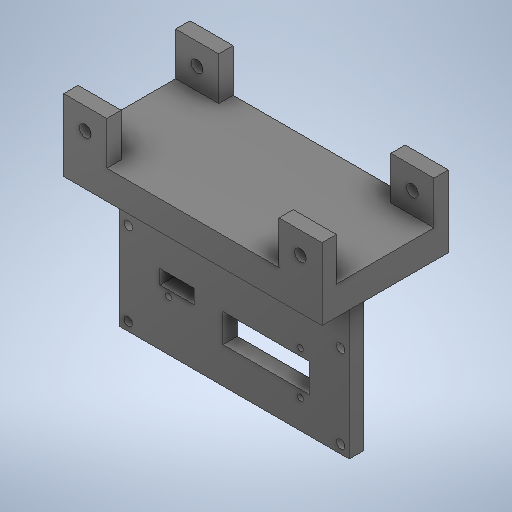
# Autodesk Inventor part: rail_top
Saved by Autodesk Inventor 2026.2 (Build 302298010, 298A)
## iProperties
Created: 2026-05-03
Part Number: rail_top
Material: ABS Plastic
Document SubType Name: Modeling
Designer: chris
Density: 1.06 g/cm^3
Appearance: Smooth - White
Author: chris
Autodesk Inventor part; units mm, degrees
ref_plane "YZ Plane" through (0, 0, 0) normal (1, 0, 0) x (0, 1, 0)
ref_plane "XZ Plane" through (0, 0, 0) normal (0, 1, 0) x (-1, 0, 0)
ref_plane "XY Plane" through (0, 0, 0) normal (0, 0, 1) x (1, 0, 0)
sketch "Sketch1" plane through (0, 0, 0) normal (0, 1, 0) x (-1, 0, 0)
  line L0 (45, 22) -> (-45, 22)
  line L1 (-45, 22) -> (-45, -22)
  line L2 (-45, -22) -> (45, -22)
  line L3 (45, -22) -> (45, 22)
  line L4 (45, 22) -> (-45, -22) construction
  line L5 (-45, 22) -> (45, -22) construction
  point P0 (0, 0)
  dimension "d0" = 90
  dimension "d1" = 44
  constraints: 12 end point, 2 midpoint, 2 parallel, 1 horizontal, 1 perpendicular
  measures "d0" distance of L2.end L1.end
  measures "d1" distance of L1.end L0.end
extrude "Extrusion1" add sketch "Sketch1" along normal blind 10
sketch "Sketch2" plane through (0, 10, 0) normal (0, 1, 0) x (1, 0, 0)
  line L0 (45, -22) -> (30, -22)
  line L1 (30, -22) -> (30, -17)
  line L2 (30, -17) -> (45, -17)
  line L3 (45, -17) -> (45, -22)
  line L4 (45, 17) -> (30, 17)
  line L5 (30, 17) -> (30, 22)
  line L6 (30, 22) -> (45, 22)
  line L7 (45, 22) -> (45, 17)
  line L8 (-45, -22) -> (-30, -22)
  line L9 (-30, -22) -> (-30, -17)
  line L10 (-30, -17) -> (-45, -17)
  line L11 (-45, -17) -> (-45, -22)
  line L12 (-45, 17) -> (-30, 17)
  line L13 (-30, 17) -> (-30, 22)
  line L14 (-30, 22) -> (-45, 22)
  line L15 (-45, 22) -> (-45, 17)
  line L16 (-45, 22) -> (-45, -22) projected
  line L17 (-45, -22) -> (45, -22) projected
  line L18 (45, 22) -> (-45, 22) projected
  line L19 (45, -22) -> (45, 22) projected
  point P0 (0, 0)
  dimension "d4" = 5
  dimension "d5" = 5
  dimension "d6" = 5
  dimension "d7" = 5
  dimension "d8" = 15
  dimension "d9" = 15
  dimension "d10" = 15
  dimension "d11" = 15
  constraints: 32 end point, 8 collinear, 8 parallel, 4 horizontal, 4 perpendicular
  measures "d4" distance of L2.end L0.start
  measures "d5" distance of L6.end L4.start
  measures "d6" distance of L12.end L13.end
  measures "d7" distance of L8.end L9.end
  measures "d8" distance of L0.start L0.end
  measures "d9" distance of L5.end L6.end
  measures "d10" distance of L12.start L12.end
  measures "d11" distance of L9.end L10.end
extrude "Extrusion2" add sketch "Sketch2" along normal blind 15 contours L0 L1 L2 L3 | L8 L11 L10 L9 | L4 L5 L6 L7 | L15 L14 L13 L12
sketch "Sketch3" plane through (-45, 0, 22) normal (0, 0, 1) x (1, 0, 0)
  circle A0 centre (82.5, 17.5) radius 2.05
  circle A1 centre (7.5, 17.5) radius 2.05
  line L0 (75, 25) -> (90, 25) projected
  line L1 (90, 0) -> (90, 25) projected
  line L2 (0, 25) -> (15, 25) projected
  line L3 (15, 10) -> (15, 25) projected
  point P0 (45, 0)
  point P1 (15, 17.5)
  dimension "d14" = 4.1
  dimension "d15" = 4.1
  dimension "d16" = 7.5
  dimension "d17" = 7.5
  dimension "d18" = 7.5
  dimension "d19" = 7.5
  constraints: 2 centre point, 1 midpoint
  measures "d14" diameter of A0
  measures "d15" diameter of A1
  measures "d16" distance from line of L0 A0.centre
  measures "d17" distance from line of L1 A0.centre
  measures "d18" distance from line of L2 A1.centre
  measures "d19" distance of point (15, 17.5) A1.centre
extrude "Extrusion3" cut sketch "Sketch3" against normal through all
sketch "Sketch6" plane through (0, 0, 0) normal (0, -1, 0) x (1, 0, 0)
  line L0 (-7.5, -7.5) -> (7.5, -7.5)
  line L1 (7.5, -7.5) -> (7.5, 7.5)
  line L2 (7.5, 7.5) -> (-7.5, 7.5)
  line L3 (-7.5, 7.5) -> (-7.5, -7.5)
  line L4 (-7.5, -7.5) -> (7.5, 7.5) construction
  line L5 (7.5, -7.5) -> (-7.5, 7.5) construction
  point P0 (0, 0)
  dimension "d27" = 15
  dimension "d28" = 15
  constraints: 12 end point, 2 midpoint, 2 parallel, 1 horizontal, 1 perpendicular
  measures "d27" distance of L2.end L1.end
  measures "d28" distance of L1.end L0.end
extrude "Extrusion5" add sketch "Sketch6" along normal blind 15
sketch "Sketch7" plane through (7.5, 0, -7.5) normal (0, 0, -1) x (-1, 0, 0)
  circle A0 centre (7.5, -7.5) radius 4.5
  line L0 (-37.5, 0) -> (52.5, 0) projected
  line L1 (0, 0) -> (0, -15) projected
  point P0 (7.5, 0)
  dimension "d31" = 9
  dimension "d32" = 7.5
  dimension "d33" = 7.5
  constraints: 1 centre point
  measures "d31" diameter of A0
  measures "d32" distance from line of A0.centre L0
  measures "d33" distance from line of L1 A0.centre
extrude "Extrusion6" cut sketch "Sketch7" against normal through all
sketch "Sketch8" plane through (-7.5, 0, 7.5) normal (0, 0, 1) x (1, 0, 0)
  line L0 (47.5, 0) -> (-32.5, 0)
  line L1 (-32.5, 0) -> (-32.5, -50)
  line L2 (-32.5, -50) -> (47.5, -50)
  line L3 (47.5, -50) -> (47.5, 0)
  line L4 (-37.5, 0) -> (52.5, 0) projected
  line L5 (0, 0) -> (0, -15) projected
  line L6 (15, -15) -> (0, -15) projected
  line L7 (15, 0) -> (15, -15) projected
  circle A0 centre (7.5, -7.5) radius 4.5 projected
  line L8 (0, 0) -> (15, 0) projected
  line L9 (0, 0) -> (0, -15) projected
  line L10 (15, -15) -> (0, -15) projected
  line L11 (15, 0) -> (15, -15) projected
  point P0 (7.5, 0)
  point P1 (7.5, 0)
  dimension "d36" = 50
  dimension "d37" = 80
  dimension "d38" = 40
  constraints: 8 end point, 2 parallel, 1 collinear, 1 horizontal, 1 midpoint, 1 perpendicular
  measures "d36" distance of L0.end L1.end
  measures "d37" distance of L1.end L2.end
  measures "d38" distance from line of point (7.5, 0) L1
extrude "Extrusion7" add sketch "Sketch8" against normal blind 5 contours L3 L2 L1 L0 L5 L6 L7
sketch "Sketch10" plane through (-7.5, 0, 2.5) normal (0, 0, -1) x (-1, 0, 0)
  circle A0 centre (29.5, -47) radius 1.5
  circle A1 centre (-44.5, -47) radius 1.5
  circle A2 centre (29.5, -18) radius 1.5
  circle A3 centre (-44.5, -18) radius 1.5
  line L0 (-47.5, -50) -> (32.5, -50) projected
  line L1 (-47.5, 0) -> (-47.5, -50) projected
  line L2 (32.5, -50) -> (32.5, 0) projected
  point P0 (-7.5, 0)
  dimension "d58" = 3
  dimension "d59" = 3
  dimension "d60" = 3
  dimension "d61" = 3
  dimension "d62" = 3
  dimension "d63" = 3
  dimension "d64" = 3
  dimension "d65" = 3
  dimension "d66" = 29
  dimension "d67" = 29
  dimension "d68" = 3
  dimension "d69" = 3
  constraints: 4 centre point
  measures "d58" diameter of A0
  measures "d59" diameter of A1
  measures "d60" diameter of A2
  measures "d61" diameter of A3
  measures "d62" distance from line of L0 A1.centre
  measures "d63" distance from line of L1 A1.centre
  measures "d64" distance from line of A0.centre L0
  measures "d65" distance from line of L2 A0.centre
  measures "d66" distance of A3.centre A1.centre
  measures "d67" distance of A2.centre A0.centre
  measures "d68" distance from line of L1 A3.centre
  measures "d69" distance from line of L2 A2.centre
extrude "Extrusion9" cut sketch "Sketch10" against normal blind 5
sketch "Sketch11" plane through (-7.5, 0, 2.5) normal (0, 0, -1) x (-1, 0, 0)
  circle A0 centre (-30.5, -40) radius 1.05
  circle A1 centre (15.5, -32.5) radius 1.05
  circle A2 centre (-30.5, -25) radius 1.05
  line L0 (-47.5, 0) -> (-47.5, -50) projected
  line L1 (-47.5, -50) -> (32.5, -50) projected
  point P0 (-7.5, 0)
  dimension "d75" = 2.1
  dimension "d76" = 2.1
  dimension "d77" = 2.1
  dimension "d78" = 46
  dimension "d79" = 7.5
  dimension "d80" = 7.5
  dimension "d81" = 17
  dimension "d82" = 0
  dimension "d83" = 10
  constraints: 3 centre point
  measures "d75" diameter of A0
  measures "d76" diameter of A1
  measures "d77" diameter of A2
  measures "d78" horizontal distance of A1.centre A0.centre
  measures "d79" vertical distance of A1.centre A0.centre
  measures "d80" vertical distance of A1.centre A2.centre
  measures "d81" distance from line of L0 A0.centre
  measures "d82" horizontal distance of A0.centre A2.centre
  measures "d83" distance from line of L1 A0.centre
extrude "Extrusion10" cut sketch "Sketch11" against normal through all
sketch "Sketch12" plane through (-7.5, 0, 2.5) normal (0, 0, -1) x (-1, 0, 0)
  line L0 (-3.5, -37.5) -> (-33.5, -37.5)
  line L1 (-33.5, -37.5) -> (-33.5, -27.5)
  line L2 (-33.5, -27.5) -> (-3.5, -27.5)
  line L3 (-3.5, -27.5) -> (-3.5, -37.5)
  line L4 (0, -15) -> (-15, -15) projected
  line L5 (-47.5, 0) -> (-47.5, -50) projected
  point P0 (-7.5, 0)
  dimension "d86" = 30
  dimension "d87" = 10
  dimension "d88" = 12.5
  dimension "d89" = 14
  constraints: 8 end point, 2 parallel, 1 horizontal, 1 perpendicular
  measures "d86" distance of L0.start L0.end
  measures "d87" distance of L2.end L0.start
  measures "d88" distance between parallel lines of L4 L2
  measures "d89" distance between parallel lines of L5 L1
extrude "Extrusion11" cut sketch "Sketch12" against normal blind 10
sketch "Sketch13" plane through (-7.5, 0, 2.5) normal (0, 0, -1) x (-1, 0, 0)
  line L0 (18.5, -30.5) -> (6.5, -30.5)
  line L1 (6.5, -30.5) -> (6.5, -25.5)
  line L2 (6.5, -25.5) -> (18.5, -25.5)
  line L3 (18.5, -25.5) -> (18.5, -30.5)
  circle A0 centre (15.5, -32.5) radius 1.05 projected
  line L4 (-3.5, -27.5) -> (-3.5, -37.5) projected
  point P0 (-7.5, 0)
  dimension "d92" = 5
  dimension "d93" = 2
  dimension "d94" = 3
  dimension "d97" = 12
  constraints: 8 end point, 2 parallel, 1 horizontal, 1 perpendicular
  measures "d92" distance of L2.end L0.start
  measures "d93" distance from line of L0 A0.centre
  measures "d94" distance from line of L3 A0.centre
  measures "d97" distance of L1.end L2.end
extrude "Extrusion12" cut sketch "Sketch13" against normal through all contours L0 L1 L2 L3
body "Solid1"
